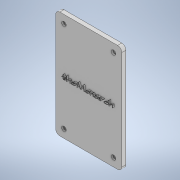
# Autodesk Inventor part: theMonarchPCBLid
Saved by Autodesk Inventor 2020 (Build 240168000, 168)
## iProperties
Created: 2020-10-14
Part Number: theMonarchPCBLid
Material: Generic
Document SubType Name: Modeling
Designer: s4393944
Density: 1 g/cm^3
Appearance: Default
Author: s4393944
Autodesk Inventor part; units mm, degrees
ref_plane "YZ Plane" through (0, 0, 0) normal (1, 0, 0) x (0, 1, 0)
ref_plane "XZ Plane" through (0, 0, 0) normal (0, 1, 0) x (-1, 0, 0)
ref_plane "XY Plane" through (0, 0, 0) normal (0, 0, 1) x (1, 0, 0)
sketch "Sketch1" plane through (0, 0, 0) normal (0, 0, 1) x (1, 0, 0)
  line L0 (40, -65) -> (-40, -65)
  line L1 (-40, -65) -> (-40, 65)
  line L2 (-40, 65) -> (40, 65)
  line L3 (40, 65) -> (40, -65)
  line L4 (40, -65) -> (-40, 65) construction
  line L5 (-40, -65) -> (40, 65) construction
  point P0 (0, 0)
  dimension "d0" = 80
  dimension "d1" = 130
  constraints: 12 end point, 2 midpoint, 2 parallel, 1 horizontal, 1 perpendicular
  measures "d0" distance of L1.end L2.end
  measures "d1" distance of L0.end L1.end
extrude "Extrusion1" add sketch "Sketch1" along normal blind 5
sketch "Sketch2" plane through (0, 0, 5) normal (0, 0, 1) x (1, 0, 0)
  circle A0 centre (-30, 55) radius 1.6
  circle A1 centre (30, 55) radius 1.6
  circle A2 centre (30, -55) radius 1.6
  circle A3 centre (-30, -55) radius 1.6
  line L0 (40, 65) -> (-40, 65) projected
  line L1 (-40, -65) -> (40, -65) projected
  point P0 (0, 0)
  dimension "d4" = 3.2
  dimension "d6" = 3.2
  dimension "d7" = 3.2
  dimension "d8" = 3.2
  dimension "d9" = 10
  dimension "d10" = 10
  dimension "d11" = 10
  dimension "d12" = 10
  dimension "d13" = 30
  dimension "d14" = 30
  dimension "d15" = 30
  dimension "d16" = 30
  constraints: 4 centre point
  measures "d4" diameter of A0
  measures "d6" diameter of A1
  measures "d7" diameter of A2
  measures "d8" diameter of A3
  measures "d9" distance from line of L0 A0.centre
  measures "d10" distance from line of L0 A1.centre
  measures "d11" distance from line of L1 A3.centre
  measures "d12" distance from line of L1 A2.centre
  measures "d13" horizontal distance of point (0, 0) A0.centre
  measures "d14" horizontal distance of point (0, 0) A1.centre
  measures "d15" horizontal distance of point (0, 0) A3.centre
  measures "d16" horizontal distance of point (0, 0) A2.centre
hole "Hole1" at (-30, 55, 5) at (30, 55, 5) at (30, -55, 5) at (-30, -55, 5) direction (0, 0, -1) diameter 3.2 end through all
sketch "Sketch3" plane through (0, 0, 5) normal (0, 0, 1) x (1, 0, 0)
  circle A0 centre (-30, 55) radius 1.6
  circle A1 centre (30, 55) radius 1.6
  circle A2 centre (30, -55) radius 1.6
  circle A3 centre (-30, -55) radius 1.6
  line L0 (40, 65) -> (-40, 65)
  line L1 (-40, -65) -> (40, -65)
  point P0 (0, 0)
  point P1 (0, 0)
  dimension "d24" = 3.2
  dimension "d25" = 3.2
  dimension "d26" = 3.2
  dimension "d27" = 3.2
  dimension "d28" = 10
  dimension "d29" = 10
  dimension "d30" = 10
  dimension "d31" = 10
  dimension "d32" = 30
  dimension "d33" = 30
  dimension "d34" = 30
  dimension "d35" = 30
  constraints: 4 centre point, 4 end point
  measures "d24" diameter of A0
  measures "d25" diameter of A1
  measures "d26" diameter of A2
  measures "d27" diameter of A3
  measures "d28" distance from line of L0 A0.centre
  measures "d29" distance from line of L0 A1.centre
  measures "d30" distance from line of L1 A3.centre
  measures "d31" distance from line of L1 A2.centre
  measures "d32" horizontal distance of point (0, 0) A0.centre
  measures "d33" horizontal distance of point (0, 0) A1.centre
  measures "d34" horizontal distance of point (0, 0) A3.centre
  measures "d35" horizontal distance of point (0, 0) A2.centre
hole "Hole2" at (-30, 55, 5) at (30, 55, 5) at (30, -55, 5) at (-30, -55, 5) direction (0, 0, -1) diameter 3.2 end through all counterbore diameter 5.5 counterbore depth 2
fillet "Fillet1" radius 5 4 edges at (40, -65, 2.5) (-40, -65, 2.5) (40, 65, 2.5) (-40, 65, 2.5)
sketch "Sketch4" plane through (0, 0, 5) normal (0, 0, 1) x (1, 0, 0)
  line L0 (-30.3235, 4.2502) -> (31.8444, 4.2502) construction
  line L1 (31.8444, 4.2502) -> (31.8444, -9.5284) construction
  line L2 (31.8444, -9.5284) -> (-30.3235, -9.5284) construction
  line L3 (-30.3235, -9.5284) -> (-30.3235, 4.2502) construction
  spline S0 degree 2 poles (-25.3016, -0.2158) (-25.5324, -0.6634) (-26.1448, -1.0449) knots 0 0 0 1 1 1
  spline S1 degree 2 poles (-26.1448, -1.0449) (-26.9645, -1.6056) (-27.7654, -1.7704) knots 0 0 0 1 1 1
  spline S2 degree 2 poles (-27.7654, -1.7704) (-28.1281, -1.8458) (-28.4061, -1.8458) knots 0 0 0 1 1 1
  spline S3 degree 2 poles (-28.4061, -1.8458) (-28.9997, -1.8458) (-29.207, -1.4784) knots 0 0 0 1 1 1
  spline S4 degree 2 poles (-29.207, -1.4784) (-29.2965, -1.3182) (-29.2965, -0.9036) knots 0 0 0 1 1 1
  line L4 (-29.2965, -0.9036) -> (-29.2965, 0.8253)
  line L5 (-29.2965, 0.8253) -> (-30.8417, 0.4861)
  line L6 (-30.8417, 0.4861) -> (-30.8417, 0.8677)
  line L7 (-30.8417, 0.8677) -> (-29.2965, 1.2022)
  line L8 (-29.2965, 1.2022) -> (-29.2965, 3.4493)
  line L9 (-29.2965, 3.4493) -> (-28.6982, 3.4493)
  line L10 (-28.6982, 3.4493) -> (-28.6982, 1.3247)
  line L11 (-28.6982, 1.3247) -> (-26.5311, 1.8052)
  line L12 (-26.5311, 1.8052) -> (-26.5311, 1.4283)
  line L13 (-26.5311, 1.4283) -> (-28.6982, 0.9478)
  line L14 (-28.6982, 0.9478) -> (-28.6982, -0.9036)
  spline S5 degree 2 poles (-28.6982, -0.9036) (-28.6982, -1.2617) (-28.6887, -1.2805) knots 0 0 0 1 1 1
  spline S6 degree 2 poles (-28.6887, -1.2805) (-28.6322, -1.4642) (-28.3354, -1.4642) knots 0 0 0 1 1 1
  spline S7 degree 2 poles (-28.3354, -1.4642) (-28.1752, -1.4642) (-27.9491, -1.4171) knots 0 0 0 1 1 1
  spline S8 degree 2 poles (-27.9491, -1.4171) (-27.2943, -1.2758) (-26.6442, -0.8754) knots 0 0 0 1 1 1
  spline S9 degree 2 poles (-26.6442, -0.8754) (-26.0742, -0.4796) (-25.881, -0.2158) knots 0 0 0 1 1 1
  line L15 (-25.881, -0.2158) -> (-25.3016, -0.2158)
  line L16 (-20.4257, -1.8458) -> (-21.024, -1.8458)
  line L17 (-21.024, -1.8458) -> (-21.024, 0.7641)
  spline S10 degree 2 poles (-21.024, 0.7641) (-21.024, 1.075) (-21.0381, 1.1174) knots 0 0 0 1 1 1
  spline S11 degree 2 poles (-21.0381, 1.1174) (-21.0805, 1.2729) (-21.3019, 1.2729) knots 0 0 0 1 1 1
  spline S12 degree 2 poles (-21.3019, 1.2729) (-21.7024, 1.2729) (-22.6351, 0.8347) knots 0 0 0 1 1 1
  spline S13 degree 2 poles (-22.6351, 0.8347) (-23.714, 0.3165) (-24.4253, -0.4231) knots 0 0 0 1 1 1
  line L18 (-24.4253, -0.4231) -> (-24.4253, -1.8835)
  line L19 (-24.4253, -1.8835) -> (-25.0236, -1.8835)
  line L20 (-25.0236, -1.8835) -> (-25.0236, -0.5126)
  line L21 (-25.0236, -0.5126) -> (-25.1885, -0.5267)
  spline S14 degree 2 poles (-25.1885, -0.5267) (-25.1225, -0.3524) (-25.0236, -0.2582) knots 0 0 0 1 1 1
  line L22 (-25.0236, -0.2582) -> (-25.0236, 4.1748)
  line L23 (-25.0236, 4.1748) -> (-24.4253, 4.1748)
  line L24 (-24.4253, 4.1748) -> (-24.4253, 0.1705)
  spline S15 degree 2 poles (-24.4253, 0.1705) (-23.8082, 0.7594) (-23.0262, 1.1315) knots 0 0 0 1 1 1
  spline S16 degree 2 poles (-23.0262, 1.1315) (-21.7495, 1.7487) (-21.1135, 1.7487) knots 0 0 0 1 1 1
  spline S17 degree 2 poles (-21.1135, 1.7487) (-20.5953, 1.7487) (-20.4681, 1.3435) knots 0 0 0 1 1 1
  spline S18 degree 2 poles (-20.4681, 1.3435) (-20.4257, 1.2305) (-20.4257, 0.7641) knots 0 0 0 1 1 1
  line L25 (-20.4257, 0.7641) -> (-20.4257, -1.8458)
  spline S19 degree 2 poles (-13.9246, 0.9855) (-14.2308, 0.5521) (-15.4321, 0.2647) knots 0 0 0 1 1 1
  spline S20 degree 2 poles (-15.4321, 0.2647) (-16.4167, 0.0339) (-17.1421, 0.0339) knots 0 0 0 1 1 1
  spline S21 degree 2 poles (-17.1421, 0.0339) (-17.3683, 0.0339) (-17.4813, 0.1234) knots 0 0 0 1 1 1
  line L26 (-17.4813, 0.1234) -> (-16.9867, 0.4861)
  spline S22 degree 2 poles (-16.9867, 0.4861) (-16.9867, 0.4202) (-16.8124, 0.4202) knots 0 0 0 1 1 1
  spline S23 degree 2 poles (-16.8124, 0.4202) (-16.2895, 0.4202) (-15.531, 0.6227) knots 0 0 0 1 1 1
  spline S24 degree 2 poles (-15.531, 0.6227) (-14.6689, 0.8536) (-14.4899, 1.108) knots 0 0 0 1 1 1
  spline S25 degree 2 poles (-14.4899, 1.108) (-14.4145, 1.2257) (-14.4145, 1.2823) knots 0 0 0 1 1 1
  spline S26 degree 2 poles (-14.4145, 1.2823) (-14.4145, 1.4377) (-14.9186, 1.4377) knots 0 0 0 1 1 1
  spline S27 degree 2 poles (-14.9186, 1.4377) (-15.4886, 1.4377) (-16.4449, 1.2399) knots 0 0 0 1 1 1
  spline S28 degree 2 poles (-16.4449, 1.2399) (-17.0621, 1.1174) (-17.7828, 0.6651) knots 0 0 0 1 1 1
  spline S29 degree 2 poles (-17.7828, 0.6651) (-18.6591, 0.1092) (-18.8428, -0.5079) knots 0 0 0 1 1 1
  spline S30 degree 2 poles (-18.8428, -0.5079) (-18.8852, -0.6398) (-18.8852, -0.7576) knots 0 0 0 1 1 1
  spline S31 degree 2 poles (-18.8852, -0.7576) (-18.8852, -1.436) (-17.7028, -1.436) knots 0 0 0 1 1 1
  spline S32 degree 2 poles (-17.7028, -1.436) (-16.2989, -1.436) (-14.5181, -0.5267) knots 0 0 0 1 1 1
  line L27 (-14.5181, -0.5267) -> (-14.113, -0.7529)
  spline S33 degree 2 poles (-14.113, -0.7529) (-16.0822, -1.8175) (-17.764, -1.8175) knots 0 0 0 1 1 1
  spline S34 degree 2 poles (-17.764, -1.8175) (-18.5413, -1.8175) (-19.4835, -1.2899) (-19.4835, -0.7717) knots 0 0 0 1 2 2 2
  spline S35 degree 2 poles (-19.4835, -0.7717) (-19.4835, -0.6162) (-19.4317, -0.4231) knots 0 0 0 1 1 1
  spline S36 degree 2 poles (-19.4317, -0.4231) (-19.2197, 0.3118) (-18.2115, 0.8818) knots 0 0 0 1 1 1
  spline S37 degree 2 poles (-18.2115, 0.8818) (-17.3494, 1.4424) (-16.6569, 1.5885) knots 0 0 0 1 1 1
  spline S38 degree 2 poles (-16.6569, 1.5885) (-15.7665, 1.7675) (-14.9798, 1.7675) knots 0 0 0 1 1 1
  spline S39 degree 2 poles (-14.9798, 1.7675) (-13.8162, 1.7675) (-13.8162, 1.3011) knots 0 0 0 1 1 1
  spline S40 degree 2 poles (-13.8162, 1.3011) (-13.8162, 1.1504) (-13.9246, 0.9855) knots 0 0 0 1 1 1
  line L28 (-3.2306, -1.8458) -> (-3.8289, -1.8458)
  line L29 (-3.8289, -1.8458) -> (-5.0397, 3.4022)
  line L30 (-5.0397, 3.4022) -> (-7.7673, -1.8081)
  line L31 (-7.7673, -1.8081) -> (-8.2196, -1.8081)
  line L32 (-8.2196, -1.8081) -> (-10.7399, 3.3457)
  line L33 (-10.7399, 3.3457) -> (-12.0213, -1.8081)
  line L34 (-12.0213, -1.8081) -> (-12.6055, -1.8081)
  line L35 (-12.6055, -1.8081) -> (-11.0744, 4.2125)
  line L36 (-11.0744, 4.2125) -> (-10.5986, 4.2125)
  line L37 (-10.5986, 4.2125) -> (-7.9934, -1.0968)
  line L38 (-7.9934, -1.0968) -> (-5.1621, 4.2502)
  line L39 (-5.1621, 4.2502) -> (-4.6722, 4.2502)
  line L40 (-4.6722, 4.2502) -> (-3.2306, -1.8458)
  spline S41 degree 2 poles (2.8324, 0.1045) (2.2671, -0.6963) (1.8242, -1.0449) knots 0 0 0 1 1 1
  spline S42 degree 2 poles (1.8242, -1.0449) (0.9339, -1.7327) (-0.4323, -1.8552) knots 0 0 0 1 1 1
  spline S43 degree 2 poles (-0.4323, -1.8552) (-0.5737, -1.8694) (-0.7008, -1.8694) knots 0 0 0 1 1 1
  spline S44 degree 2 poles (-0.7008, -1.8694) (-1.4405, -1.8694) (-1.8739, -1.5113) knots 0 0 0 1 1 1
  spline S45 degree 2 poles (-1.8739, -1.5113) (-2.2884, -1.1721) (-2.2884, -0.6398) knots 0 0 0 1 1 1
  spline S46 degree 2 poles (-2.2884, -0.6398) (-2.2884, -0.3242) (-2.1189, 0.0244) knots 0 0 0 1 1 1
  spline S47 degree 2 poles (-2.1189, 0.0244) (-1.3745, 1.4848) (1.4002, 1.6968) knots 0 0 0 1 1 1
  spline S48 degree 2 poles (1.4002, 1.6968) (2.1116, 1.7487) (2.5639, 1.433) knots 0 0 0 1 1 1
  spline S49 degree 2 poles (2.5639, 1.433) (3.0114, 1.108) (3.0114, 0.6369) knots 0 0 0 1 1 1
  spline S50 degree 2 poles (3.0114, 0.6369) (3.0114, 0.3542) (2.8324, 0.1045) knots 0 0 0 1 1 1
  spline S51 degree 2 poles (2.3142, 0.2883) (2.4272, 0.4531) (2.4272, 0.6698) knots 0 0 0 1 1 1
  spline S52 degree 2 poles (2.4272, 0.6698) (2.4272, 0.9619) (2.2058, 1.1409) knots 0 0 0 1 1 1
  spline S53 degree 2 poles (2.2058, 1.1409) (1.9279, 1.3576) (1.4709, 1.32) knots 0 0 0 1 1 1
  spline S54 degree 2 poles (1.4709, 1.32) (-0.8704, 1.1409) (-1.6006, -0.1734) knots 0 0 0 1 1 1
  spline S55 degree 2 poles (-1.6006, -0.1734) (-1.7043, -0.4231) (-1.7043, -0.7058) knots 0 0 0 1 1 1
  spline S56 degree 2 poles (-1.7043, -0.7058) (-1.7043, -1.0497) (-1.4687, -1.2522) knots 0 0 0 1 1 1
  spline S57 degree 2 poles (-1.4687, -1.2522) (-1.2049, -1.4878) (-0.7291, -1.4878) knots 0 0 0 1 1 1
  spline S58 degree 2 poles (-0.7291, -1.4878) (-0.6161, -1.4878) (-0.536, -1.4831) knots 0 0 0 1 1 1
  spline S59 degree 2 poles (-0.536, -1.4831) (0.6606, -1.3747) (1.4144, -0.767) knots 0 0 0 1 1 1
  spline S60 degree 2 poles (1.4144, -0.767) (1.763, -0.4843) (2.3142, 0.2883) knots 0 0 0 1 1 1
  line L41 (7.7177, -1.8458) -> (7.1194, -1.8458)
  line L42 (7.1194, -1.8458) -> (7.1194, 0.0339)
  spline S61 degree 2 poles (7.1194, 0.0339) (7.1194, 0.6369) (7.0864, 0.7923) knots 0 0 0 1 1 1
  spline S62 degree 2 poles (7.0864, 0.7923) (6.9875, 1.2257) (6.6765, 1.2257) knots 0 0 0 1 1 1
  spline S63 degree 2 poles (6.6765, 1.2257) (6.6153, 1.2257) (6.5446, 1.2069) knots 0 0 0 1 1 1
  spline S64 degree 2 poles (6.5446, 1.2069) (5.381, 0.9572) (4.0714, -0.1404) knots 0 0 0 1 1 1
  line L43 (4.0714, -0.1404) -> (4.0714, -1.8458)
  line L44 (4.0714, -1.8458) -> (3.4731, -1.8458)
  line L45 (3.4731, -1.8458) -> (3.4731, -0.3666)
  line L46 (3.4731, -0.3666) -> (3.2045, -0.3666)
  spline S65 degree 2 poles (3.2045, -0.3666) (3.2705, -0.1923) (3.4731, -0.0321) knots 0 0 0 1 1 1
  line L47 (3.4731, -0.0321) -> (3.4731, 1.7392)
  line L48 (3.4731, 1.7392) -> (4.0714, 1.7392)
  line L49 (4.0714, 1.7392) -> (4.0714, 0.3542)
  spline S66 degree 2 poles (4.0714, 0.3542) (5.4234, 1.4472) (6.5117, 1.6639) knots 0 0 0 1 1 1
  spline S67 degree 2 poles (6.5117, 1.6639) (6.7048, 1.6968) (6.8367, 1.6968) knots 0 0 0 1 1 1
  spline S68 degree 2 poles (6.8367, 1.6968) (7.4633, 1.6968) (7.6329, 1.0938) knots 0 0 0 1 1 1
  spline S69 degree 2 poles (7.6329, 1.0938) (7.7177, 0.8018) (7.7177, 0.0386) knots 0 0 0 1 1 1
  line L50 (7.7177, 0.0386) -> (7.7177, -1.8458)
  spline S70 degree 2 poles (14.6616, -0.3477) (14.5392, -0.6115) (14.5109, -0.6351) knots 0 0 0 1 1 1
  line L51 (14.5109, -0.6351) -> (14.5109, -1.8458)
  line L52 (14.5109, -1.8458) -> (13.8937, -1.8458)
  line L53 (13.8937, -1.8458) -> (13.8937, -0.9225)
  spline S71 degree 2 poles (13.8937, -0.9225) (13.1965, -1.2522) (11.9999, -1.5302) knots 0 0 0 1 1 1
  spline S72 degree 2 poles (11.9999, -1.5302) (10.6338, -1.8458) (9.7198, -1.8458) knots 0 0 0 1 1 1
  spline S73 degree 2 poles (9.7198, -1.8458) (8.3254, -1.8458) (8.4432, -1.158) knots 0 0 0 1 1 1
  spline S74 degree 2 poles (8.4432, -1.158) (8.5703, -0.3571) (10.8693, 0.1705) knots 0 0 0 1 1 1
  spline S75 degree 2 poles (10.8693, 0.1705) (12.5181, 0.5521) (13.8937, 0.6416) knots 0 0 0 1 1 1
  line L54 (13.8937, 0.6416) -> (13.8937, 0.9431)
  spline S76 degree 2 poles (13.8937, 0.9431) (13.8937, 1.1127) (13.3002, 1.4189) (12.9044, 1.4189) knots 0 0 0 1 2 2 2
  spline S77 degree 2 poles (12.9044, 1.4189) (12.5323, 1.4189) (11.2697, 1.2116) knots 0 0 0 1 1 1
  spline S78 degree 2 poles (11.2697, 1.2116) (9.9742, 1.0043) (9.8988, 0.8771) knots 0 0 0 1 1 1
  line L55 (9.8988, 0.8771) -> (9.3005, 0.8771)
  spline S79 degree 2 poles (9.3005, 0.8771) (9.3241, 1.2022) (10.5301, 1.4566) knots 0 0 0 1 1 1
  spline S80 degree 2 poles (10.5301, 1.4566) (11.543, 1.6733) (12.6124, 1.7863) knots 0 0 0 1 1 1
  spline S81 degree 2 poles (12.6124, 1.7863) (12.7584, 1.8005) (12.8903, 1.8005) knots 0 0 0 1 1 1
  spline S82 degree 2 poles (12.8903, 1.8005) (13.5027, 1.8005) (14.5109, 1.2964) (14.5109, 0.9478) knots 0 0 0 1 2 2 2
  line L56 (14.5109, 0.9478) -> (14.5109, 0.585)
  spline S83 degree 2 poles (14.5109, 0.585) (14.5109, 0.6133) (14.6145, 0.5379) (14.6145, 0.4531) knots 0 0 0 1 2 2 2
  line L57 (14.6145, 0.4531) -> (14.5109, 0.3495)
  line L58 (14.5109, 0.3495) -> (14.5109, -0.3242)
  line L59 (14.5109, -0.3242) -> (14.6616, -0.3477)
  line L60 (13.8937, -0.4938) -> (13.8937, 0.2788)
  spline S84 degree 2 poles (13.8937, 0.2788) (12.5747, 0.1658) (11.1708, -0.1357) knots 0 0 0 1 1 1
  spline S85 degree 2 poles (11.1708, -0.1357) (9.1922, -0.5786) (9.0273, -1.1769) knots 0 0 0 1 1 1
  spline S86 degree 2 poles (9.0273, -1.1769) (8.9095, -1.5113) (9.7905, -1.5113) knots 0 0 0 1 1 1
  spline S87 degree 2 poles (9.7905, -1.5113) (10.7044, -1.5113) (12.1413, -1.1345) knots 0 0 0 1 1 1
  spline S88 degree 2 poles (12.1413, -1.1345) (13.4933, -0.7764) (13.8937, -0.4938) knots 0 0 0 1 1 1
  spline S89 degree 2 poles (19.66, 1.2776) (19.3019, 1.3153) (19.0617, 1.3153) knots 0 0 0 1 1 1
  spline S90 degree 2 poles (19.0617, 1.3153) (17.3422, 1.3153) (16.1739, 0.26) knots 0 0 0 1 1 1
  line L61 (16.1739, 0.26) -> (16.1739, -1.8458)
  line L62 (16.1739, -1.8458) -> (15.5756, -1.8458)
  line L63 (15.5756, -1.8458) -> (15.5756, 0.1893)
  line L64 (15.5756, 0.1893) -> (15.3683, 0.1893)
  spline S91 degree 2 poles (15.3683, 0.1893) (15.4719, 0.3919) (15.5756, 0.4767) knots 0 0 0 1 1 1
  line L65 (15.5756, 0.4767) -> (15.5756, 1.7016)
  line L66 (15.5756, 1.7016) -> (16.1739, 1.7016)
  line L67 (16.1739, 1.7016) -> (16.1739, 0.8489)
  spline S92 degree 2 poles (16.1739, 0.8489) (17.2998, 1.7016) (18.9251, 1.7016) knots 0 0 0 1 1 1
  spline S93 degree 2 poles (18.9251, 1.7016) (19.2171, 1.7016) (19.66, 1.6639) knots 0 0 0 1 1 1
  line L68 (19.66, 1.6639) -> (19.66, 1.2776)
  line L69 (25.1671, 1.4236) -> (24.7525, 1.1645)
  spline S94 degree 2 poles (24.7525, 1.1645) (24.4039, 1.287) (24.0082, 1.287) knots 0 0 0 1 1 1
  spline S95 degree 2 poles (24.0082, 1.287) (22.9906, 1.287) (20.9037, 0.1234) (20.7294, -0.5503) knots 0 0 0 1 2 2 2
  spline S96 degree 2 poles (20.7294, -0.5503) (20.7058, -0.6304) (20.7058, -0.7246) knots 0 0 0 1 1 1
  spline S97 degree 2 poles (20.7058, -0.7246) (20.7058, -1.4124) (22.1097, -1.4124) knots 0 0 0 1 1 1
  spline S98 degree 2 poles (22.1097, -1.4124) (23.4994, -1.4124) (24.7337, -0.8235) knots 0 0 0 1 1 1
  line L70 (24.7337, -0.8235) -> (25.1247, -1.0638)
  spline S99 degree 2 poles (25.1247, -1.0638) (23.7444, -1.7846) (22.1097, -1.7846) knots 0 0 0 1 1 1
  spline S100 degree 2 poles (22.1097, -1.7846) (21.2287, -1.7846) (20.7529, -1.5537) knots 0 0 0 1 1 1
  spline S101 degree 2 poles (20.7529, -1.5537) (20.1217, -1.2711) (20.1217, -0.734) knots 0 0 0 1 1 1
  spline S102 degree 2 poles (20.1217, -0.734) (20.1217, -0.6021) (20.1546, -0.4514) knots 0 0 0 1 1 1
  spline S103 degree 2 poles (20.1546, -0.4514) (20.3525, 0.3259) (22.9058, 1.6215) (24.1542, 1.6215) knots 0 0 0 1 2 2 2
  spline S104 degree 2 poles (24.1542, 1.6215) (24.7007, 1.6215) (25.1671, 1.4236) knots 0 0 0 1 1 1
  line L71 (30.7449, -1.8458) -> (30.1466, -1.8458)
  line L72 (30.1466, -1.8458) -> (30.1466, 0.7641)
  spline S105 degree 2 poles (30.1466, 0.7641) (30.1466, 1.075) (30.1325, 1.1174) knots 0 0 0 1 1 1
  spline S106 degree 2 poles (30.1325, 1.1174) (30.0901, 1.2729) (29.8687, 1.2729) knots 0 0 0 1 1 1
  spline S107 degree 2 poles (29.8687, 1.2729) (29.4682, 1.2729) (28.5355, 0.8347) knots 0 0 0 1 1 1
  spline S108 degree 2 poles (28.5355, 0.8347) (27.4566, 0.3165) (26.7453, -0.4231) knots 0 0 0 1 1 1
  line L73 (26.7453, -0.4231) -> (26.7453, -1.8835)
  line L74 (26.7453, -1.8835) -> (26.147, -1.8835)
  line L75 (26.147, -1.8835) -> (26.147, -0.5126)
  line L76 (26.147, -0.5126) -> (25.9821, -0.5267)
  spline S109 degree 2 poles (25.9821, -0.5267) (26.0481, -0.3524) (26.147, -0.2582) knots 0 0 0 1 1 1
  line L77 (26.147, -0.2582) -> (26.147, 4.1748)
  line L78 (26.147, 4.1748) -> (26.7453, 4.1748)
  line L79 (26.7453, 4.1748) -> (26.7453, 0.1705)
  spline S110 degree 2 poles (26.7453, 0.1705) (27.3624, 0.7594) (28.1444, 1.1315) knots 0 0 0 1 1 1
  spline S111 degree 2 poles (28.1444, 1.1315) (29.4211, 1.7487) (30.0571, 1.7487) knots 0 0 0 1 1 1
  spline S112 degree 2 poles (30.0571, 1.7487) (30.5753, 1.7487) (30.7025, 1.3435) knots 0 0 0 1 1 1
  spline S113 degree 2 poles (30.7025, 1.3435) (30.7449, 1.2305) (30.7449, 0.7641) knots 0 0 0 1 1 1
  line L80 (30.7449, 0.7641) -> (30.7449, -1.8458)
  point P0 (0, 0)
  constraints: 2 other
emboss "Emboss1" sketch "Sketch4" operation add depth 2 direction (0, 0, -1)
body "Solid1"
